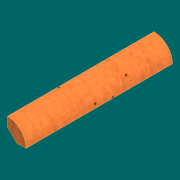
# Autodesk Inventor part: sideMoulding
Saved by Autodesk Inventor 2016 SP1 (Build 200210100, 210)
## iProperties
Created: 2016-04-01
Part Number: sideMoulding
Material: Wood (Cherry)
Document SubType Name: Modeling
Designer: sawai
Density: 0.63 g/cm^3
Appearance: Cherry - Natural Low Gloss
Author: sawai
Autodesk Inventor part; units mm, degrees
ref_plane "YZ Plane" through (0, 0, 0) normal (1, 0, 0) x (0, 1, 0)
ref_plane "XZ Plane" through (0, 0, 0) normal (0, 1, 0) x (-1, 0, 0)
ref_plane "XY Plane" through (0, 0, 0) normal (0, 0, 1) x (1, 0, 0)
sketch "Sketch1" plane through (0, 0, 0) normal (1, 0, 0) x (0, 1, 0)
  line L0 (-6.35, 6.35) -> (6.35, 6.35)
  line L1 (6.35, 6.35) -> (6.35, -6.35)
  line L2 (6.35, -6.35) -> (-6.35, -6.35)
  line L3 (-6.35, -6.35) -> (-6.35, 6.35)
  line L4 (-6.35, 6.35) -> (6.35, -6.35) construction
  line L5 (6.35, 6.35) -> (-6.35, -6.35) construction
  point P0 (0, 0)
  dimension "d0" = 12.7
  dimension "d1" = 12.7
  constraints: 12 end point, 2 midpoint, 2 parallel, 1 horizontal, 1 perpendicular
  measures "d0" distance of L1.end L2.end
  measures "d1" distance of L0.end L1.end
extrude "Extrusion1" add sketch "Sketch1" along normal mid plane 100
chamfer "Chamfer1" distance 6.35 angle 45 1 edges at (0, -6.35, -6.35)
fillet "Fillet1" radius 12.7 1 edges at (0, 6.35, 6.35)
equation "\"d0\" = facingThickness"
equation "\"d1\" = facingThickness"
equation "\"d2\" = depth"
equation "\"d4\" = 0.5 * facingThickness"
equation "\"d7\" = facingThickness"
equation "\"mppcMountThickness\" = 6.35"
equation "\"depth\" = 100"
equation "\"facingThickness\" = 12.7"
equation "\"facingGasketThickness\" = 1.5875"
body "Solid1"
